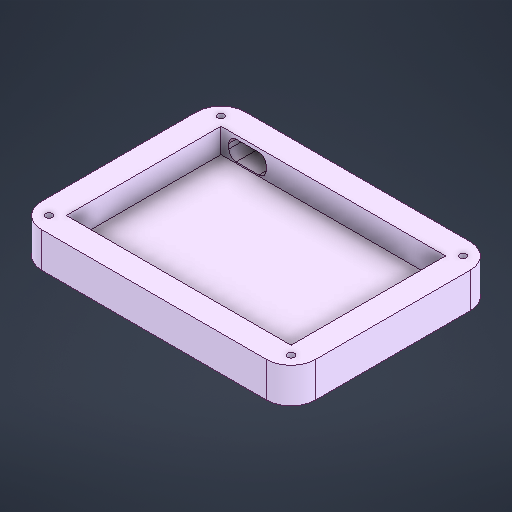
# Autodesk Inventor part: Bottom
Saved by Autodesk Inventor 2026.2 (Build 302298000, 298)
## iProperties
Created: 2026-02-15
Part Number: Bottom
Material: Generic
Document SubType Name: Modeling
Designer: bh
Density: 1 g/cm^3
Appearance: Default
Author: bh
Autodesk Inventor part; units mm, degrees
ref_plane "YZ Plane" through (0, 0, 0) normal (1, 0, 0) x (0, 1, 0)
ref_plane "XZ Plane" through (0, 0, 0) normal (0, 1, 0) x (-1, 0, 0)
ref_plane "XY Plane" through (0, 0, 0) normal (0, 0, 1) x (1, 0, 0)
sketch "Sketch1" plane through (0, 0, 0) normal (0, 1, 0) x (-1, 0, 0)
  line L0 (0, 0) -> (-91.4, 0)
  line L1 (-91.4, 0) -> (-91.4, -62.9)
  line L2 (-91.4, -62.9) -> (0, -62.9)
  line L3 (0, -62.9) -> (0, 0)
  line L4 (10, 10) -> (-101.4, 10)
  line L5 (-101.4, 10) -> (-101.4, -72.9)
  line L6 (-101.4, -72.9) -> (10, -72.9)
  line L7 (10, -72.9) -> (10, 10)
  dimension "d0" = 91.4
  dimension "d1" = 62.9
  dimension "d4" = 10
  constraints: 16 end point, 4 parallel, 2 perpendicular, 1 horizontal, 3 other
  measures "d0" distance of L2.end L1.end
  measures "d1" distance of L1.end L0.end
  measures "d4" distance between parallel lines of L3 L7
extrude "Extrusion1" add sketch "Sketch1" along normal blind 10
sketch "Sketch2" plane through (0, 0, 0) normal (0, -1, 0) x (1, 0, 0)
  line L0 (101.4, 10) -> (101.4, -72.9) projected
  line L1 (101.4, -72.9) -> (-10, -72.9) projected
  line L2 (-10, -72.9) -> (-10, 10) projected
  line L3 (-10, 10) -> (101.4, 10) projected
  point P0 (0, 0)
extrude "Extrusion2" add sketch "Sketch2" along normal blind 0.3
fillet "Fillet1" radius 10 4 edges at (-10, 4.85, -72.9) (101.4, 4.85, -72.9) (101.4, 4.85, 10) (-10, 4.85, 10)
sketch "Sketch5" plane through (0, -0.3, 0) normal (0, -1, 0) x (1, 0, 0)
  arc A0 (0, 10) -> (-10, 0) centre (0, 0) ccw projected
  line L0 (-10, 0) -> (-10, -62.9) projected
  arc A1 (-10, -62.9) -> (0, -72.9) centre (0, -62.9) ccw projected
  line L1 (0, -72.9) -> (91.4, -72.9) projected
  arc A2 (91.4, -72.9) -> (101.4, -62.9) centre (91.4, -62.9) ccw projected
  line L2 (101.4, -62.9) -> (101.4, 0) projected
  arc A3 (101.4, 0) -> (91.4, 10) centre (91.4, 0) ccw projected
  line L3 (91.4, 10) -> (0, 10) projected
  line L4 (91.4, 0) -> (0, 0) projected
  line L5 (91.4, -62.9) -> (91.4, 0) projected
  line L6 (0, -62.9) -> (91.4, -62.9) projected
  line L7 (0, 0) -> (0, -62.9) projected
  line L8 (-2.5102, 4.5608) -> (-1.9699, 5.1011)
  circle A4 centre (-3.5355, 3.5355) radius 1.45
  line L9 (45.7, 0) -> (45.7, -31.45)
  line L10 (93.635, 4.1768) -> (91.995, 4.9855)
  circle A5 centre (94.9355, 3.5355) radius 1.45
  line L11 (95.8901, -65.4809) -> (96.3855, -64.9855)
  line L12 (-4.4901, -65.4809) -> (-4.9855, -64.9855)
  circle A6 centre (-3.5355, -66.4355) radius 1.35
  circle A7 centre (94.9355, -66.4355) radius 1.35
  line L13 (0, 0) -> (-2.5102, 2.5102)
  line L14 (-4.5608, 4.5608) -> (-7.0711, 7.0711)
  line L15 (91.4, 0) -> (93.9102, 2.5102)
  line L16 (95.9608, 4.5608) -> (98.4711, 7.0711)
  line L17 (91.4, -62.9) -> (93.9809, -65.4809)
  line L18 (95.8901, -67.3901) -> (98.4711, -69.9711)
  line L19 (0, -62.9) -> (-2.5809, -65.4809)
  line L20 (-4.4901, -67.3901) -> (-7.0711, -69.9711)
  constraints: 26 end point, 16 point on circle, 4 centre point, 4 perpendicular, 1 midpoint, 1 parallel
extrude "Extrusion3" cut sketch "Sketch5" against normal blind 16 contours A4 | A5 | A6 | A7
sketch "Sketch6" plane through (0, -0.3, 0) normal (0, -1, 0) x (1, 0, 0)
  circle A0 centre (94.9355, -66.4355) radius 1.35 projected
  circle A1 centre (94.9355, 3.5355) radius 1.45 projected
  circle A2 centre (-3.5355, -66.4355) radius 1.35 projected
  circle A3 centre (-3.5355, 3.5355) radius 1.45 projected
  arc A4 (0, 10) -> (-10, 0) centre (0, 0) ccw projected
  line L0 (-10, 0) -> (-10, -62.9) projected
  arc A5 (-10, -62.9) -> (0, -72.9) centre (0, -62.9) ccw projected
  line L1 (0, -72.9) -> (91.4, -72.9) projected
  arc A6 (91.4, -72.9) -> (101.4, -62.9) centre (91.4, -62.9) ccw projected
  line L2 (101.4, -62.9) -> (101.4, 0) projected
  arc A7 (101.4, 0) -> (91.4, 10) centre (91.4, 0) ccw projected
  line L3 (91.4, 10) -> (0, 10) projected
  circle A8 centre (-3.5355, -66.4355) radius 2.85
  circle A9 centre (-3.5355, 3.5355) radius 2.95
  circle A10 centre (94.9355, 3.5355) radius 2.95
  circle A11 centre (94.9355, -66.4355) radius 2.85
  point P0 (0, 0)
  dimension "d16" = 1.5
  dimension "d17" = 1.5
  dimension "d18" = 1.5
  dimension "d19" = 1.5
  constraints: 4 centre point
  measures "d16" radial gap between concentric circles of A2 A8
  measures "d17" radial gap between concentric circles of A3 A9
  measures "d18" radial gap between concentric circles of A1 A10
  measures "d19" radial gap between concentric circles of A0 A11
extrude "Extrusion4" add sketch "Sketch6" along normal blind 4 contours L3 A7 L2 A6 L1 A5 L0 A4
sketch "Sketch7" plane through (91.4, 10, -72.9) normal (0, 0, -1) x (-1, 0, 0)
  line L0 (88.212, -2.095) -> (88.212, -9.4812)
  line L1 (88.212, -9.4812) -> (72.9957, -9.4812)
  line L2 (72.9957, -9.4812) -> (72.9957, -2.095)
  line L3 (88.212, -2.095) -> (88.212, -3.345)
  line L4 (72.9957, -3.345) -> (72.9957, -2.095)
  line L5 (88.212, -9.4812) -> (72.9957, -9.4812)
  line L6 (72.9957, -9.4812) -> (72.9957, -1.4812)
  line L7 (72.9957, -1.4812) -> (88.212, -1.4812)
  line L8 (88.212, -1.4812) -> (88.212, -9.4812)
  point P0 (91.4, -10)
  dimension "d24" = 1.25
  constraints: 18 end point, 4 parallel, 1 horizontal, 1 perpendicular, 1 point on line
  measures "d24" distance of L3.start L3.end
extrude "Extrusion5" cut sketch "Sketch7" against normal blind 44.15
fillet "Fillet2" radius 3 4 edges at (18.4043, 0.5188, -67.9) (3.188, 0.5188, -67.9) (18.4043, 8.5188, -67.9) (3.188, 8.5188, -67.9)
body "Solid1"
